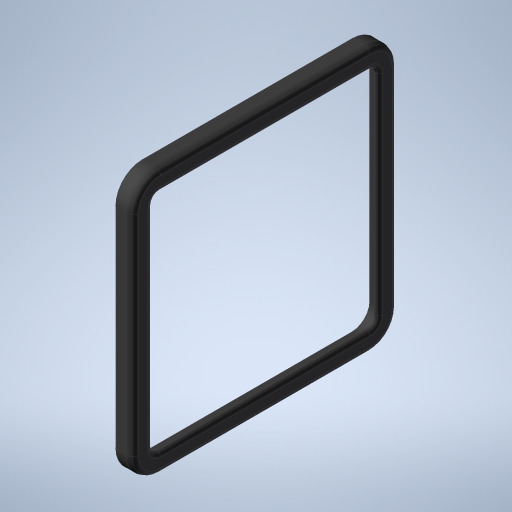
# Autodesk Inventor part: DiffuserRetainer
Saved by Autodesk Inventor 2023 (Build 270158000, 158)
## iProperties
Created: 2026-01-19
Part Number: DiffuserRetainer
Material: Generic
Document SubType Name: Modeling
Designer: DanAr
Density: 1 g/cm^3
Appearance: Default
Author: DanAr
Autodesk Inventor part; units mm, degrees
ref_plane "YZ Plane" through (0, 0, 0) normal (1, 0, 0) x (0, 1, 0)
ref_plane "XZ Plane" through (0, 0, 0) normal (0, 1, 0) x (-1, 0, 0)
ref_plane "XY Plane" through (0, 0, 0) normal (0, 0, 1) x (1, 0, 0)
sketch "Sketch1" plane through (0, 0, 0) normal (1, 0, 0) x (0, 1, 0)
  line L0 (0, 0) -> (160, 0)
  line L1 (160, 0) -> (160, -160)
  line L2 (160, -160) -> (0, -160)
  line L3 (0, -160) -> (0, 0)
  line L4 (0, 0) -> (5, 0)
  line L5 (5, 0) -> (5, -5)
  line L6 (5, -5) -> (0, -5)
  line L7 (0, -5) -> (0, 0)
  line L8 (5, -5) -> (155, -5)
  line L9 (155, -5) -> (155, -155)
  line L10 (155, -155) -> (5, -155)
  line L11 (5, -155) -> (5, -5)
  dimension "d0" = 160
  dimension "d1" = 160
  dimension "d2" = 5
  dimension "d3" = 5
  dimension "d4" = 150
  dimension "d5" = 150
  constraints: 24 end point, 6 parallel, 3 horizontal, 3 perpendicular
  measures "d0" distance of L0.end L1.end
  measures "d1" distance of L1.end L2.end
  measures "d2" distance of L4.end L5.end
  measures "d3" distance of L5.end L6.end
  measures "d4" distance of L8.end L9.end
  measures "d5" distance of L9.end L10.end
extrude "Extrusion1" add sketch "Sketch1" along normal blind 10
sketch "Sketch2" plane through (10, 0, 0) normal (1, 0, 0) x (0, 0, -1)
  line L0 (5, 155) -> (155, 155) projected
  line L1 (5, 155) -> (10, 155)
  line L2 (10, 155) -> (10, 150)
  line L3 (10, 150) -> (5, 150)
  line L4 (5, 150) -> (5, 155)
  line L5 (10, 150) -> (150, 150)
  line L6 (150, 150) -> (150, 10)
  line L7 (150, 10) -> (10, 10)
  line L8 (10, 10) -> (10, 150)
  line L9 (160, 0) -> (160, 160) projected
  line L10 (0, 160) -> (160, 160)
  line L11 (160, 160) -> (160, 0)
  line L12 (160, 0) -> (0, 0)
  line L13 (0, 0) -> (0, 160)
  point P0 (0, 0)
  dimension "d8" = 5
  dimension "d9" = 5
  dimension "d10" = 140
  dimension "d11" = 140
  constraints: 24 end point, 6 parallel, 3 horizontal, 3 perpendicular
  measures "d8" distance of L1.end L2.end
  measures "d9" distance of L2.end L3.end
  measures "d10" distance of L5.end L6.end
  measures "d11" distance of L6.end L7.end
extrude "Extrusion2" add sketch "Sketch2" along normal blind 4 contours L0 L2 L3 L4 | L12 L13 L10 L9
fillet "Fillet1" radius 10 4 edges at (5, 5, -155) (5, 155, -155) (5, 155, -5) (5, 5, -5)
fillet "Fillet2" radius 5 4 edges at (12, 10, -150) (12, 150, -150) (12, 10, -10) (12, 150, -10)
sketch "Sketch3" plane through (0, 0, 0) normal (-1, 0, 0) x (0, 0, 1)
  line L0 (-160, 160) -> (0, 160) projected
  line L1 (-160, 160) -> (0, 160) construction
  line L2 (-160, 150) -> (0, 150)
  line L3 (0, 170) -> (-160, 170)
  arc A0 (-160, 170) -> (-160, 150) centre (-160, 160) ccw
  arc A1 (0, 150) -> (0, 170) centre (0, 160) ccw
  line L4 (0, 160) -> (0, 0) projected
  line L5 (0, 0) -> (0, 160) construction
  line L6 (10, 0) -> (10, 160)
  line L7 (-10, 160) -> (-10, 0)
  arc A2 (-10, 0) -> (10, 0) centre (0, 0) ccw
  arc A3 (10, 160) -> (-10, 160) centre (0, 160) ccw
  line L8 (-160, 0) -> (-160, 160) projected
  line L9 (0, 0) -> (-160, 0) construction
  line L10 (0, 10) -> (-160, 10)
  line L11 (-160, -10) -> (0, -10)
  arc A4 (0, -10) -> (0, 10) centre (0, 0) ccw
  arc A5 (-160, 10) -> (-160, -10) centre (-160, 0) ccw
  line L12 (0, 0) -> (-160, 0) projected
  line L13 (-160, 0) -> (-160, 160) construction
  line L14 (-150, 0) -> (-150, 160)
  line L15 (-170, 160) -> (-170, 0)
  arc A6 (-170, 0) -> (-150, 0) centre (-160, 0) ccw
  arc A7 (-150, 160) -> (-170, 160) centre (-160, 160) ccw
  line L16 (-160, 160) -> (0, 160)
  line L17 (0, 160) -> (0, 0)
  line L18 (0, 0) -> (-160, 0)
  line L19 (-160, 0) -> (-160, 160)
  point P0 (-80, 160)
  point P1 (0, 80)
  point P2 (-80, 0)
  point P3 (-160, 80)
  point P4 (-170, 0)
  dimension "d16" = 10
  constraints: 40 end point, 16 point on circle, 16 tangent, 8 centre point, 8 equal length, 4 midpoint, 3 perpendicular, 1 horizontal
  measures "d16" radius of A1
extrude "Extrusion3" add sketch "Sketch3" against normal up to surface (14 mm away) contours L8 A0 A7 L0 | A7 L3 A3 L0 | L8 A5 L15 A0 | A3 A1 L4 L0 | L8 L12 A6 A5 | A1 L6 A4 L4 | L12 A2 L11 A6 | A4 A2 L12 L4
sketch "Sketch4" plane through (0, 0, 0) normal (-1, 0, 0) x (0, 0, 1)
  line L0 (-15, 150) -> (-145, 150) projected
  line L1 (-80, 150) -> (-80, 10)
  line L2 (-145, 10) -> (-15, 10) projected
  line L3 (-155.5, 4.5) -> (-4.5, 4.5)
  line L4 (-4.5, 4.5) -> (-4.5, 155.5)
  line L5 (-4.5, 155.5) -> (-155.5, 155.5)
  line L6 (-155.5, 155.5) -> (-155.5, 4.5)
  line L7 (-155.5, 4.5) -> (-4.5, 155.5) construction
  line L8 (-4.5, 4.5) -> (-155.5, 155.5) construction
  arc A0 (-145, 150) -> (-150, 145) centre (-145, 145) ccw projected
  circle A1 centre (-145, 145) radius 10.5
  arc A2 (-5, 145) -> (-15, 155) centre (-15, 145) ccw projected
  circle A3 centre (-15, 145) radius 10.5
  arc A4 (-15, 10) -> (-10, 15) centre (-15, 15) ccw projected
  circle A5 centre (-15, 15) radius 10.5
  arc A6 (-150, 15) -> (-145, 10) centre (-145, 15) ccw projected
  circle A7 centre (-145, 15) radius 10.5
  point P0 (0, 0)
  point P1 (-80, 80)
  point P2 (-4.5, 145)
  point P3 (-15, 155.5)
  point P4 (-145, 155.5)
  point P5 (-155.5, 145)
  point P6 (-155.5, 15)
  point P7 (-145, 4.5)
  point P8 (-15, 4.5)
  point P9 (-4.5, 15)
  dimension "d19" = 151
  dimension "d20" = 151
  constraints: 14 end point, 5 midpoint, 4 centre point, 4 coincident, 4 tangent, 2 parallel, 1 horizontal, 1 perpendicular
  measures "d19" distance of L4.end L5.end
  measures "d20" distance of L3.end L4.end
extrude "Extrusion4" cut sketch "Sketch4" against normal up to surface (10 mm away) contours A3 L4 A5 L2 L1 L0 | L0 A1 L5 A3 | A3 | L1 L2 A7 L6 A1 L0 | A1 | L2 A5 L3 A7 | A5 | A7
sketch "Sketch6" plane through (0, 0, 0) normal (-1, 0, 0) x (0, 0, 1)
  arc A0 (-145, 150) -> (-150, 145) centre (-145, 145) ccw projected
  circle A1 centre (-155.5, 155.5) radius 1.5 projected
  circle A2 centre (-155.5, 155.5) radius 1.5 projected
  arc A3 (-145, 155.5) -> (-155.5, 145) centre (-145, 145) ccw projected
  line L0 (-155.5, 155.5) -> (-145, 145)
  line L1 (-145, 145) -> (-155.5, 155.5)
  line L2 (-155.5, 155.5) -> (-158.5309, 158.5309)
  circle A4 centre (-145, 145) radius 17
  arc A5 (-10, 145) -> (-15, 150) centre (-15, 145) ccw projected
  line L3 (-145, 145) -> (-15, 145) construction
  line L4 (-145, 162) -> (-15, 162)
  line L5 (-15, 128) -> (-145, 128)
  arc A6 (-145, 162) -> (-145, 128) centre (-145, 145) ccw
  arc A7 (-15, 128) -> (-15, 162) centre (-15, 145) ccw
  arc A8 (-150, 15) -> (-145, 10) centre (-145, 15) ccw projected
  line L6 (-145, 145) -> (-145, 15) construction
  line L7 (-128, 145) -> (-128, 15)
  line L8 (-162, 15) -> (-162, 145)
  arc A9 (-128, 145) -> (-162, 145) centre (-145, 145) ccw
  arc A10 (-162, 15) -> (-128, 15) centre (-145, 15) ccw
  arc A11 (-15, 10) -> (-10, 15) centre (-15, 15) ccw projected
  line L9 (-145, 15) -> (-15, 15) construction
  line L10 (-145, 32) -> (-15, 32)
  line L11 (-15, -2) -> (-145, -2)
  arc A12 (-145, 32) -> (-145, -2) centre (-145, 15) ccw
  arc A13 (-15, -2) -> (-15, 32) centre (-15, 15) ccw
  line L12 (-15, 15) -> (-15, 145) construction
  line L13 (2, 15) -> (2, 145)
  line L14 (-32, 145) -> (-32, 15)
  arc A14 (-32, 15) -> (2, 15) centre (-15, 15) ccw
  arc A15 (2, 145) -> (-32, 145) centre (-15, 145) ccw
  line L15 (-180.2133, 180.2133) -> (20.1008, 180.2133)
  line L16 (20.1008, 180.2133) -> (20.1008, -29.1514)
  line L17 (20.1008, -29.1514) -> (-180.2133, -29.1514)
  line L18 (-180.2133, -29.1514) -> (-180.2133, 180.2133)
  point P0 (0, 0)
  point P1 (-80, 145)
  point P2 (-145, 80)
  point P3 (-80, 15)
  point P4 (-15, 80)
  point P5 (2, 145)
  point P6 (2, 15)
  point P7 (-145, -2)
  point P8 (-162, 145)
  point P9 (-145, 162)
  dimension "d26" = 10.5
  dimension "d27" = 10.5
  dimension "d28" = 34
  dimension "d38" = 164
  dimension "d39" = 17
  dimension "d43" = 17
  dimension "d44" = 17
  constraints: 46 end point, 16 point on circle, 16 tangent, 9 centre point, 7 equal length, 4 midpoint, 4 perpendicular, 2 horizontal, 1 coincident, 1 concentric, 1 point on line
  measures "d26" horizontal distance of A0.centre A1.centre
  measures "d27" horizontal distance of A0.centre A1.centre
  measures "d28" diameter of A4
  measures "d38" distance between parallel lines of L11 L4
  measures "d39" radius of A15
  measures "d43" radius of A13
  measures "d44" radius of A9
extrude "Extrusion6" cut sketch "Sketch6" against normal blind 30 contours L15 L16 L17 L18
fillet "Fillet3" radius 6 4 edges at (14, 157.0208, -2.9792) (14, 2.9792, -2.9792) (14, 2.9792, -157.0208) (14, 157.0208, -157.0208)
chamfer "Chamfer1" distance 3 angle 45 4 edges at (14, 150, -80) (14, 80, -10) (14, 10, -80) (14, 80, -150)
fillet "Fillet4" radius 2 8 edges at (14, 150.6569, -150.6569) (14, 153, -80) (14, 150.6569, -9.3431) (14, 80, -7) (14, 9.3431, -9.3431) (14, 7, -80) (14, 9.3431, -150.6569) (14, 80, -153)
fillet "Fillet5" radius 1 8 edges at (11, 80, -150) (11, 11.4645, -148.5355) (11, 10, -80) (11, 11.4645, -11.4645) (11, 80, -10) (11, 148.5355, -11.4645) (11, 150, -80) (11, 148.5355, -148.5355)
fillet "Fillet6" radius 1 12 edges at (0, 152.4246, -152.4246) (0, 155.5, -80) (0, 152.4246, -7.5754) (0, 80, -4.5) (0, 7.5754, -7.5754) (0, 4.5, -80) (0, 7.5754, -152.4246) (0, 80, -155.5) (0, 2.9792, -157.0208) (0, 2.9792, -2.9792) (0, 157.0208, -2.9792) (0, 157.0208, -157.0208)
sketch "Sketch8" plane through (14, 0, 0) normal (1, 0, 0) x (0, 0, -1)
  line L0 (162, 15) -> (162, 145) projected
  line L1 (-2, 145) -> (-2, 15) projected
  line L2 (15, -2) -> (145, -2) projected
  line L3 (145, 162) -> (15, 162) projected
  line L4 (145, 155.5) -> (15, 155.5) projected
  point P0 (0, 0)
  dimension "d40" = 164
  dimension "d41" = 164
  dimension "d42" = 6.5
  measures "d40" distance between parallel lines of L0 L1
  measures "d41" distance between parallel lines of L2 L3
  measures "d42" distance between parallel lines of L4 L3
sketch "Sketch9" plane through (0, 0, 0) normal (-1, 0, 0) x (0, 0, 1)
  line L0 (-15, 150) -> (-145, 150) projected
  line L1 (-80, 150) -> (-80, 10)
  line L2 (-145, 10) -> (-15, 10) projected
  line L3 (-154.75, 5.25) -> (-5.25, 5.25)
  line L4 (-5.25, 5.25) -> (-5.25, 154.75)
  line L5 (-5.25, 154.75) -> (-154.75, 154.75)
  line L6 (-154.75, 154.75) -> (-154.75, 5.25)
  line L7 (-154.75, 5.25) -> (-5.25, 154.75) construction
  line L8 (-5.25, 5.25) -> (-154.75, 154.75) construction
  circle A0 centre (-154.75, 154.75) radius 1.6
  circle A1 centre (-5.25, 154.75) radius 1.6
  circle A2 centre (-154.75, 5.25) radius 1.6
  circle A3 centre (-5.25, 5.25) radius 1.6
  point P0 (0, 0)
  point P1 (-145, 145)
  point P2 (-15, 15)
  point P3 (-80, 80)
  dimension "d48" = 149.5
  dimension "d49" = 149.5
  dimension "d50" = 3.2
  constraints: 14 end point, 5 midpoint, 4 centre point, 4 coincident, 2 parallel, 1 horizontal, 1 perpendicular
  measures "d48" distance of L4.end L5.end
  measures "d49" distance of L3.end L4.end
  measures "d50" diameter of A0
extrude "Extrusion7" cut sketch "Sketch9" against normal blind 10 contours L6 A2 L3 | L3 A2 L6 | A3 L4 L3 | L3 L4 A3 | A0 L5 L6 | L6 L5 A0 | A1 L5 L4 | L4 L5 A1
sketch "Sketch10" plane through (8, 15, 2) normal (0, 0, 1) x (1, 0, 0)
  line L0 (6, 0) -> (6, 130) projected
  line L1 (-8, 130) -> (-8, 0) projected
  line L2 (0, 130) -> (0, 0) projected
  point P0 (-8, -15)
  dimension "d53" = 14
  dimension "d54" = 8
  measures "d53" distance between parallel lines of L0 L1
  measures "d54" distance between parallel lines of L2 L1
sketch "Sketch11" plane through (10, 0, 0) normal (-1, 0, 0) x (0, 0, 1)
  line L0 (-145, 10) -> (-15, 10) projected
  line L1 (-15, 150) -> (-145, 150) projected
  line L2 (-15, 4.5) -> (-145, 4.5) projected
  line L3 (-145, 155.5) -> (-15, 155.5) projected
  line L4 (-80, 150) -> (-80, 10)
  line L5 (-7, 7) -> (-153, 7)
  line L6 (-153, 7) -> (-153, 153)
  line L7 (-153, 153) -> (-7, 153)
  line L8 (-7, 153) -> (-7, 7)
  line L9 (-7, 7) -> (-153, 153) construction
  line L10 (-153, 7) -> (-7, 153) construction
  point P0 (0, 0)
  point P1 (-80, 80)
  dimension "d55" = 140
  dimension "d56" = 151
  dimension "d57" = 146
  dimension "d58" = 146
  constraints: 14 end point, 5 midpoint, 2 parallel, 1 horizontal, 1 perpendicular
  measures "d55" distance between parallel lines of L0 L1
  measures "d56" distance between parallel lines of L2 L3
  measures "d57" distance of L6.end L7.end
  measures "d58" distance of L5.end L6.end
chamfer "Chamfer2" distance 0.3 angle 45 4 edges at (0, 154.75, -6.85) (0, 154.75, -156.35) (0, 5.25, -156.35) (0, 5.25, -6.85)
sketch "Sketch17" plane through (14, 0, 0) normal (1, 0, 0) x (0, 0, -1)
  line L0 (-21.1254, 169.9507) -> (180.25, 169.9507)
  line L1 (180.25, 169.9507) -> (180.25, -9.9186)
  line L2 (180.25, -9.9186) -> (-21.1254, -9.9186)
  line L3 (-21.1254, -9.9186) -> (-21.1254, 169.9507)
  point P0 (0, 0)
  constraints: 8 end point, 2 parallel, 1 horizontal, 1 perpendicular
extrude "Extrusion8" cut sketch "Sketch17" against normal blind 1.5
fillet "Fillet7" radius 3 16 edges at (12.5, 159.9686, -80) (12.5, 155.5844, -155.5844) (12.5, 80, -159.9686) (12.5, 4.4156, -155.5844) (12.5, 0.0314, -80) (12.5, 4.4156, -4.4156) (12.5, 80, -0.0314) (12.5, 155.5844, -4.4156) (12.5, 80, -8.5) (12.5, 10.4038, -10.4038) (12.5, 8.5, -80) (12.5, 10.4038, -149.5962) (12.5, 80, -151.5) (12.5, 149.5962, -149.5962) (12.5, 151.5, -80) (12.5, 149.5962, -10.4038)
sketch "Sketch18" plane through (0, 0, 0) normal (-1, 0, 0) x (0, 0, 1)
  line L0 (-183.9063, 166.801) -> (38.1322, 166.801)
  line L1 (38.1322, 166.801) -> (38.1322, -27.1199)
  line L2 (38.1322, -27.1199) -> (-183.9063, -27.1199)
  line L3 (-183.9063, -27.1199) -> (-183.9063, 166.801)
  point P0 (0, 0)
  constraints: 8 end point, 2 parallel, 1 horizontal, 1 perpendicular
extrude "Extrusion9" cut sketch "Sketch18" against normal blind 1
fillet "Fillet8" radius 1 16 edges at (1, 80, -155.5) (1, 152.4246, -152.4246) (1, 155.5, -80) (1, 152.4246, -7.5754) (1, 80, -4.5) (1, 7.5754, -7.5754) (1, 4.5, -80) (1, 7.5754, -152.4246) (1, 2.9792, -157.0208) (1, -2, -80) (1, 2.9792, -2.9792) (1, 80, 2) (1, 157.0208, -2.9792) (1, 162, -80) (1, 157.0208, -157.0208) (1, 80, -162)
chamfer "Chamfer3" distance 0.3 angle 45 4 edges at (1, 5.25, -156.35) (1, 154.75, -156.35) (1, 154.75, -6.85) (1, 5.25, -6.85)
body "Solid1"
